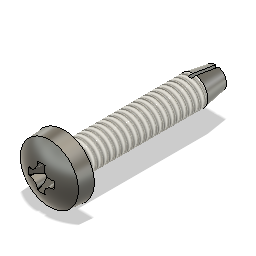
Focus Dial (Autodesk Fusion 360 archive; units mm, degrees)
design "Type I Cross Recessed Pan Head Tapping Screw ANSI B18.6.5M M2x0.4 x 10 Type D Steel Grade 2 Plain"
description: Type I Cross Recessed Pan Head Tapping Screw ANSI B18.6.5M M2x0.4 x 10 Type D
Autodesk Fusion 360 part; units mm, degrees
sketch "Sketch1" plane through (0, 0, 0) normal (0, 1, 0) x (1, 0, 0)
  line L0 (-1, 0) -> (-1, 10)
  line L1 (-1, 10) -> (0, 10)
  line L2 (0, 10) -> (0, -1.6)
  line L3 (-1, 0) -> (-2, 0)
  arc A0 (-1.9157, -0.9632) -> (0, -1.6) centre (0, 1.6) ccw
  line L4 (-2, 0) -> (-1.9157, -0.9632)
  dimension "d9" = 2
  dimension "d66" = 4
  dimension "d67" = 1.6
  dimension "d68" = 10
  dimension "d70" = 3.2
  dimension "d79" = 85
  constraint perpendicular L0 L1
  constraint collinear origin L2.end L1.end
  constraint perpendicular L0 L3
  constraint coincident origin L3
  constraint vertical L0
  constraint vertical L2
  constraint coincident L2 A0.centre
  measures "d67" vertical distance of L2.end L3.end
  measures "d68" distance of origin L1.end
  measures "d70" radius of A0
  measures "d79" angle of L3 L4
revolve "Revolve1" add sketch "Sketch1" angle 360 about axis through (0, 0, -10) along (0, 0, 1) makes body 1
ref_plane "WorkPlane1" through (0, 0, 1.6) normal (0, 0, 1) x (1, 0, 0)
sketch "Sketch7" plane through (0, 0, 1.6) normal (0, 0, 1) x (1, 0, 0)
  line L0 (-0.24, -0.91) -> (-0.24, -0.24)
  line L1 (-0.24, -0.24) -> (-0.91, -0.24)
  line L2 (-0.91, -0.24) -> (-0.91, 0)
  line L3 (-0.91, 0) -> (0, 0) construction
  line L4 (0, -0.91) -> (-0.24, -0.91)
  line L5 (0, 0) -> (0, -0.91) construction
  circle A0 centre (0, 0) radius 0.91 construction
  line L6 (0.24, -0.91) -> (0, -0.91)
  line L7 (0.24, -0.24) -> (0.24, -0.91)
  line L8 (0.91, -0.24) -> (0.24, -0.24)
  line L9 (0.91, 0) -> (0.91, -0.24)
  line L10 (0.91, 0.24) -> (0.91, 0)
  line L11 (0.24, 0.24) -> (0.91, 0.24)
  line L12 (0.24, 0.91) -> (0.24, 0.24)
  line L13 (0, 0.91) -> (0.24, 0.91)
  line L14 (-0.24, 0.91) -> (0, 0.91)
  line L15 (-0.24, 0.24) -> (-0.24, 0.91)
  line L16 (-0.91, 0.24) -> (-0.24, 0.24)
  line L17 (-0.91, 0) -> (-0.91, 0.24)
  dimension "d98" = 1.82
  dimension "d99" = 0.24
  dimension "d100" = 0.24
  dimension "d113" = 360
  constraint coincident L3.end L5.start
  constraint coincident L4.start A0
  constraint vertical L5
  constraint parallel L0 L5
  constraint perpendicular L1 L5
  constraint perpendicular L1 L2
  constraint perpendicular L3 L5
  constraint coincident L2.end A0
  constraint perpendicular L4 L5
  constraint coincident L0.end L1.start
  measures "d98" diameter of A0
  measures "d99" distance of L4.start L0.start
  measures "d100" distance of L1.end L2.end
thread "Thread1" "ISO Metric profile 2.0 M2x0.4 6g" major diameter 1.9335 minor diameter 1.478 pitch 0.4 angle 60 resizes the face on face at (-0.995, 0.0996, -3.3333) on bodies 1
extrude "Extrude4" add sketch "Sketch7" against normal blind 1.19 draft -4 separate body makes body 2
draft "Draft2" angle -30 neutral plane through (0, 0, 1.6) pull (0, 0, 1) 8 faces at (-0.1323, 0.8823, 1.2033) (0.1323, 0.8823, 1.2033) (0.8823, 0.1323, 1.2033) (0.8823, -0.1323, 1.2033) (0.1323, -0.8823, 1.2033) (-0.1323, -0.8823, 1.2033) (-0.8823, -0.1323, 1.2033) (-0.8823, 0.1323, 1.2033) on bodies 2
fillet "Fillet4" radius 0.48 4 edges at (-0.1984, -0.1984, 1.005) (0.1984, -0.1984, 1.005) (0.1984, 0.1984, 1.005) (-0.1984, 0.1984, 1.005) on bodies 2
combine "Combine1" operation cut target body 1 tool bodies 2
sketch "Sketch5" plane through (0, 0, 0) normal (0, 1, 0) x (1, 0, 0)
  line L0 (-1.02, 10) -> (-1.02, 8.2)
  line L1 (-1.02, 8.2) -> (-0.725, 10)
  line L2 (0, 10) -> (0, -1.6)
  line L3 (-1.02, 10) -> (0, 10)
  dimension "d86" = 1.02
  dimension "d88" = 1.8
  dimension "d89" = 0.725
  constraint coincident L2.start L3.end
  constraint perpendicular L2 L3
  constraint coincident L1.end L3
  constraint perpendicular L0 L3
  measures "d86" distance of origin L0
  measures "d88" vertical distance of L0.end L1.end
  measures "d89" horizontal distance of origin L1.end
revolve "Revolve2" cut sketch "Sketch5" angle 360 about axis through (0, 0, -10) along (0, 0, 1) bodies 1
sketch "Sketch6" plane through (0, 0, -10) normal (0, 0, -1) x (-1, 0, 0)
  line L0 (0, 0) -> (-0.2, 0)
  line L1 (-0.2, 0) -> (-0.2, 2)
  line L2 (-0.2, 2) -> (0, 2)
  line L3 (0, 2) -> (0, 0)
  dimension "d108" = 0.2
  dimension "d109" = 2
  constraint horizontal L0
  constraint vertical L1
  constraint horizontal L2
  constraint vertical L3
  constraint coincident L0.start L3.end
  measures "d108" distance of L1.end L2.end
  measures "d109" distance of L0.start L2.end
extrude "Extrude3" cut sketch "Sketch6" against normal blind 1.8 bodies 1
equation "d9 = adsk_nomdia"
equation "adsk_nomlen = 10.00 mm"
equation "adsk_headh = 1.60 mm"
equation "adsk_headdia = 4.00 mm"
equation "adsk_nomdia = 2.00 mm"
equation "adsk_phildia = 1.82 mm"
equation "adsk_philwidth = 0.48 mm"
equation "adsk_phildepth = 1.19 mm"
equation "d66 = adsk_headdia"
equation "d67 = adsk_headh"
equation "d68 = adsk_nomlen"
equation "d70 = adsk_headdia * 0.8"
equation "d71 = adsk_headh"
equation "adsk_startlen = 1.80 mm"
equation "adsk_pitch1 = 0.40 mm"
equation "adsk_endpointdia = 1.45 mm"
equation "d86 = adsk_nomdia * 0.51"
equation "d88 = adsk_startlen"
equation "d89 = adsk_endpointdia / 2"
equation "d98 = adsk_phildia"
equation "d99 = adsk_philwidth / 2"
equation "d100 = adsk_philwidth / 2"
equation "d108 = adsk_nomdia / 10"
equation "d109 = adsk_headdia / 2"
equation "d110 = -adsk_startlen"
equation "d114 = -adsk_phildepth"
equation "d119 = adsk_philwidth"

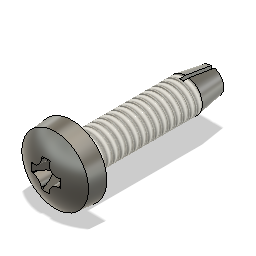
design "Type I Cross Recessed Pan Head Tapping Screw ANSI B18.6.5M M2x0.4 x 8 Type D Steel Grade 2 Plain"
description: Type I Cross Recessed Pan Head Tapping Screw ANSI B18.6.5M M2x0.4 x 8 Type D
Autodesk Fusion 360 part; units mm, degrees
sketch "Sketch1" plane through (0, 0, 0) normal (0, 1, 0) x (1, 0, 0)
  line L0 (-1, 0) -> (-1, 8)
  line L1 (-1, 8) -> (0, 8)
  line L2 (0, 8) -> (0, -1.6)
  line L3 (-1, 0) -> (-2, 0)
  arc A0 (-1.9157, -0.9632) -> (0, -1.6) centre (0, 1.6) ccw
  line L4 (-2, 0) -> (-1.9157, -0.9632)
  dimension "d9" = 2
  dimension "d66" = 4
  dimension "d67" = 1.6
  dimension "d68" = 8
  dimension "d70" = 3.2
  dimension "d79" = 85
  constraint perpendicular L0 L1
  constraint collinear origin L2.end L1.end
  constraint perpendicular L0 L3
  constraint coincident origin L3
  constraint vertical L0
  constraint vertical L2
  constraint coincident L2 A0.centre
  measures "d67" vertical distance of L2.end L3.end
  measures "d68" distance of origin L1.end
  measures "d70" radius of A0
  measures "d79" angle of L3 L4
revolve "Revolve1" add sketch "Sketch1" angle 360 about axis through (0, 0, -8) along (0, 0, 1) makes body 1
ref_plane "WorkPlane1" through (0, 0, 1.6) normal (0, 0, 1) x (1, 0, 0)
sketch "Sketch7" plane through (0, 0, 1.6) normal (0, 0, 1) x (1, 0, 0)
  line L0 (-0.24, -0.91) -> (-0.24, -0.24)
  line L1 (-0.24, -0.24) -> (-0.91, -0.24)
  line L2 (-0.91, -0.24) -> (-0.91, 0)
  line L3 (-0.91, 0) -> (0, 0) construction
  line L4 (0, -0.91) -> (-0.24, -0.91)
  line L5 (0, 0) -> (0, -0.91) construction
  circle A0 centre (0, 0) radius 0.91 construction
  line L6 (0.24, -0.91) -> (0, -0.91)
  line L7 (0.24, -0.24) -> (0.24, -0.91)
  line L8 (0.91, -0.24) -> (0.24, -0.24)
  line L9 (0.91, 0) -> (0.91, -0.24)
  line L10 (0.91, 0.24) -> (0.91, 0)
  line L11 (0.24, 0.24) -> (0.91, 0.24)
  line L12 (0.24, 0.91) -> (0.24, 0.24)
  line L13 (0, 0.91) -> (0.24, 0.91)
  line L14 (-0.24, 0.91) -> (0, 0.91)
  line L15 (-0.24, 0.24) -> (-0.24, 0.91)
  line L16 (-0.91, 0.24) -> (-0.24, 0.24)
  line L17 (-0.91, 0) -> (-0.91, 0.24)
  dimension "d98" = 1.82
  dimension "d99" = 0.24
  dimension "d100" = 0.24
  dimension "d113" = 360
  constraint coincident L3.end L5.start
  constraint coincident L4.start A0
  constraint vertical L5
  constraint parallel L0 L5
  constraint perpendicular L1 L5
  constraint perpendicular L1 L2
  constraint perpendicular L3 L5
  constraint coincident L2.end A0
  constraint perpendicular L4 L5
  constraint coincident L0.end L1.start
  measures "d98" diameter of A0
  measures "d99" distance of L4.start L0.start
  measures "d100" distance of L1.end L2.end
thread "Thread1" "ISO Metric profile 2.0 M2x0.4 6g" major diameter 1.9335 minor diameter 1.478 pitch 0.4 angle 60 resizes the face on face at (-0.995, 0.0996, -5.3333) on bodies 1
extrude "Extrude4" add sketch "Sketch7" against normal blind 1.19 draft -4 separate body makes body 2
draft "Draft2" angle -30 neutral plane through (0, 0, 1.6) pull (0, 0, 1) 8 faces at (-0.1323, 0.8823, 1.2033) (0.1323, 0.8823, 1.2033) (0.8823, 0.1323, 1.2033) (0.8823, -0.1323, 1.2033) (0.1323, -0.8823, 1.2033) (-0.1323, -0.8823, 1.2033) (-0.8823, -0.1323, 1.2033) (-0.8823, 0.1323, 1.2033) on bodies 2
fillet "Fillet4" radius 0.48 4 edges at (-0.1984, -0.1984, 1.005) (0.1984, -0.1984, 1.005) (0.1984, 0.1984, 1.005) (-0.1984, 0.1984, 1.005) on bodies 2
combine "Combine1" operation cut target body 1 tool bodies 2
sketch "Sketch5" plane through (0, 0, 0) normal (0, 1, 0) x (1, 0, 0)
  line L0 (-1.02, 8) -> (-1.02, 6.2)
  line L1 (-1.02, 6.2) -> (-0.725, 8)
  line L2 (0, 8) -> (0, -1.6)
  line L3 (-1.02, 8) -> (0, 8)
  dimension "d86" = 1.02
  dimension "d88" = 1.8
  dimension "d89" = 0.725
  constraint coincident L2.start L3.end
  constraint perpendicular L2 L3
  constraint coincident L1.end L3
  constraint perpendicular L0 L3
  measures "d86" distance of origin L0
  measures "d88" vertical distance of L0.end L1.end
  measures "d89" horizontal distance of origin L1.end
revolve "Revolve2" cut sketch "Sketch5" angle 360 about axis through (0, 0, -8) along (0, 0, 1) bodies 1
sketch "Sketch6" plane through (0, 0, -8) normal (0, 0, -1) x (-1, 0, 0)
  line L0 (0, 0) -> (-0.2, 0)
  line L1 (-0.2, 0) -> (-0.2, 2)
  line L2 (-0.2, 2) -> (0, 2)
  line L3 (0, 2) -> (0, 0)
  dimension "d108" = 0.2
  dimension "d109" = 2
  constraint horizontal L0
  constraint vertical L1
  constraint horizontal L2
  constraint vertical L3
  constraint coincident L0.start L3.end
  measures "d108" distance of L1.end L2.end
  measures "d109" distance of L0.start L2.end
extrude "Extrude3" cut sketch "Sketch6" against normal blind 1.8 bodies 1
equation "d9 = adsk_nomdia"
equation "adsk_nomlen = 8.00 mm"
equation "adsk_headh = 1.60 mm"
equation "adsk_headdia = 4.00 mm"
equation "adsk_nomdia = 2.00 mm"
equation "adsk_phildia = 1.82 mm"
equation "adsk_philwidth = 0.48 mm"
equation "adsk_phildepth = 1.19 mm"
equation "d66 = adsk_headdia"
equation "d67 = adsk_headh"
equation "d68 = adsk_nomlen"
equation "d70 = adsk_headdia * 0.8"
equation "d71 = adsk_headh"
equation "adsk_startlen = 1.80 mm"
equation "adsk_pitch1 = 0.40 mm"
equation "adsk_endpointdia = 1.45 mm"
equation "d86 = adsk_nomdia * 0.51"
equation "d88 = adsk_startlen"
equation "d89 = adsk_endpointdia / 2"
equation "d98 = adsk_phildia"
equation "d99 = adsk_philwidth / 2"
equation "d100 = adsk_philwidth / 2"
equation "d108 = adsk_nomdia / 10"
equation "d109 = adsk_headdia / 2"
equation "d110 = -adsk_startlen"
equation "d114 = -adsk_phildepth"
equation "d119 = adsk_philwidth"

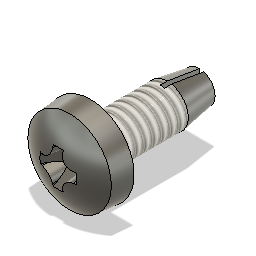
design "Type I Cross Recessed Pan Head Tapping Screw ANSI B18.6.5M M2x0.4 x 5 Type D Steel Grade 2 Plain"
description: Type I Cross Recessed Pan Head Tapping Screw ANSI B18.6.5M M2x0.4 x 5 Type D
Autodesk Fusion 360 part; units mm, degrees
sketch "Sketch1" plane through (0, 0, 0) normal (0, 1, 0) x (1, 0, 0)
  line L0 (-1, 0) -> (-1, 5)
  line L1 (-1, 5) -> (0, 5)
  line L2 (0, 5) -> (0, -1.6)
  line L3 (-1, 0) -> (-2, 0)
  arc A0 (-1.9157, -0.9632) -> (0, -1.6) centre (0, 1.6) ccw
  line L4 (-2, 0) -> (-1.9157, -0.9632)
  dimension "d9" = 2
  dimension "d66" = 4
  dimension "d67" = 1.6
  dimension "d68" = 5
  dimension "d70" = 3.2
  dimension "d79" = 85
  constraint perpendicular L0 L1
  constraint collinear origin L2.end L1.end
  constraint perpendicular L0 L3
  constraint coincident origin L3
  constraint vertical L0
  constraint vertical L2
  constraint coincident L2 A0.centre
  measures "d67" vertical distance of L2.end L3.end
  measures "d68" distance of origin L1.end
  measures "d70" radius of A0
  measures "d79" angle of L3 L4
revolve "Revolve1" add sketch "Sketch1" angle 360 about axis through (0, 0, -5) along (0, 0, 1) makes body 1
ref_plane "WorkPlane1" through (0, 0, 1.6) normal (0, 0, 1) x (1, 0, 0)
sketch "Sketch7" plane through (0, 0, 1.6) normal (0, 0, 1) x (1, 0, 0)
  line L0 (-0.24, -0.91) -> (-0.24, -0.24)
  line L1 (-0.24, -0.24) -> (-0.91, -0.24)
  line L2 (-0.91, -0.24) -> (-0.91, 0)
  line L3 (-0.91, 0) -> (0, 0) construction
  line L4 (0, -0.91) -> (-0.24, -0.91)
  line L5 (0, 0) -> (0, -0.91) construction
  circle A0 centre (0, 0) radius 0.91 construction
  line L6 (0.24, -0.91) -> (0, -0.91)
  line L7 (0.24, -0.24) -> (0.24, -0.91)
  line L8 (0.91, -0.24) -> (0.24, -0.24)
  line L9 (0.91, 0) -> (0.91, -0.24)
  line L10 (0.91, 0.24) -> (0.91, 0)
  line L11 (0.24, 0.24) -> (0.91, 0.24)
  line L12 (0.24, 0.91) -> (0.24, 0.24)
  line L13 (0, 0.91) -> (0.24, 0.91)
  line L14 (-0.24, 0.91) -> (0, 0.91)
  line L15 (-0.24, 0.24) -> (-0.24, 0.91)
  line L16 (-0.91, 0.24) -> (-0.24, 0.24)
  line L17 (-0.91, 0) -> (-0.91, 0.24)
  dimension "d98" = 1.82
  dimension "d99" = 0.24
  dimension "d100" = 0.24
  dimension "d113" = 360
  constraint coincident L3.end L5.start
  constraint coincident L4.start A0
  constraint vertical L5
  constraint parallel L0 L5
  constraint perpendicular L1 L5
  constraint perpendicular L1 L2
  constraint perpendicular L3 L5
  constraint coincident L2.end A0
  constraint perpendicular L4 L5
  constraint coincident L0.end L1.start
  measures "d98" diameter of A0
  measures "d99" distance of L4.start L0.start
  measures "d100" distance of L1.end L2.end
thread "Thread1" "ISO Metric profile 2.0 M2x0.4 6g" major diameter 1.9335 minor diameter 1.478 pitch 0.4 angle 60 resizes the face on face at (-0.9988, 0.0498, -1.6667) on bodies 1
extrude "Extrude4" add sketch "Sketch7" against normal blind 1.19 draft -4 separate body makes body 2
draft "Draft2" angle -30 neutral plane through (0, 0, 1.6) pull (0, 0, 1) 8 faces at (-0.1323, 0.8823, 1.2033) (0.1323, 0.8823, 1.2033) (0.8823, 0.1323, 1.2033) (0.8823, -0.1323, 1.2033) (0.1323, -0.8823, 1.2033) (-0.1323, -0.8823, 1.2033) (-0.8823, -0.1323, 1.2033) (-0.8823, 0.1323, 1.2033) on bodies 2
fillet "Fillet4" radius 0.48 4 edges at (-0.1984, -0.1984, 1.005) (0.1984, -0.1984, 1.005) (0.1984, 0.1984, 1.005) (-0.1984, 0.1984, 1.005) on bodies 2
combine "Combine1" operation cut target body 1 tool bodies 2
sketch "Sketch5" plane through (0, 0, 0) normal (0, 1, 0) x (1, 0, 0)
  line L0 (-1.02, 5) -> (-1.02, 3.2)
  line L1 (-1.02, 3.2) -> (-0.725, 5)
  line L2 (0, 5) -> (0, -1.6)
  line L3 (-1.02, 5) -> (0, 5)
  dimension "d86" = 1.02
  dimension "d88" = 1.8
  dimension "d89" = 0.725
  constraint coincident L2.start L3.end
  constraint perpendicular L2 L3
  constraint coincident L1.end L3
  constraint perpendicular L0 L3
  measures "d86" distance of origin L0
  measures "d88" vertical distance of L0.end L1.end
  measures "d89" horizontal distance of origin L1.end
revolve "Revolve2" cut sketch "Sketch5" angle 360 about axis through (0, 0, -5) along (0, 0, 1) bodies 1
sketch "Sketch6" plane through (0, 0, -5) normal (0, 0, -1) x (-1, 0, 0)
  line L0 (0, 0) -> (-0.2, 0)
  line L1 (-0.2, 0) -> (-0.2, 2)
  line L2 (-0.2, 2) -> (0, 2)
  line L3 (0, 2) -> (0, 0)
  dimension "d108" = 0.2
  dimension "d109" = 2
  constraint horizontal L0
  constraint vertical L1
  constraint horizontal L2
  constraint vertical L3
  constraint coincident L0.start L3.end
  measures "d108" distance of L1.end L2.end
  measures "d109" distance of L0.start L2.end
extrude "Extrude3" cut sketch "Sketch6" against normal blind 1.8 bodies 1
equation "d9 = adsk_nomdia"
equation "adsk_nomlen = 5.00 mm"
equation "adsk_headh = 1.60 mm"
equation "adsk_headdia = 4.00 mm"
equation "adsk_nomdia = 2.00 mm"
equation "adsk_phildia = 1.82 mm"
equation "adsk_philwidth = 0.48 mm"
equation "adsk_phildepth = 1.19 mm"
equation "d66 = adsk_headdia"
equation "d67 = adsk_headh"
equation "d68 = adsk_nomlen"
equation "d70 = adsk_headdia * 0.8"
equation "d71 = adsk_headh"
equation "adsk_startlen = 1.80 mm"
equation "adsk_pitch1 = 0.40 mm"
equation "adsk_endpointdia = 1.45 mm"
equation "d86 = adsk_nomdia * 0.51"
equation "d88 = adsk_startlen"
equation "d89 = adsk_endpointdia / 2"
equation "d98 = adsk_phildia"
equation "d99 = adsk_philwidth / 2"
equation "d100 = adsk_philwidth / 2"
equation "d108 = adsk_nomdia / 10"
equation "d109 = adsk_headdia / 2"
equation "d110 = -adsk_startlen"
equation "d114 = -adsk_phildepth"
equation "d119 = adsk_philwidth"
